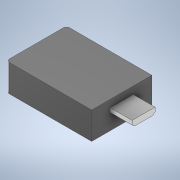
# Autodesk Inventor part: ND-105C
Saved by Autodesk Inventor 2020.2 (Build 242310000, 310)
## iProperties
Created: 2020-04-10
Part Number: ND-105C
Material: PC/ABS Plastic
Document SubType Name: Modeling
Designer: agmlego
Mass: 1.34202 g
Surface Area: 17.1017 cm^2
Volume: 3.75629 cm^3
Density: 0.357273 g/cm^3
Appearance: Smooth - Black
Author: agmlego
Autodesk Inventor part; units mm, degrees
ref_plane "YZ Plane" through (0, 0, 0) normal (1, 0, 0) x (0, 1, 0)
ref_plane "XZ Plane" through (0, 0, 0) normal (0, 1, 0) x (-1, 0, 0)
ref_plane "XY Plane" through (0, 0, 0) normal (0, 0, 1) x (1, 0, 0)
sketch "Sketch1" plane through (0, 0, 0) normal (0, 1, 0) x (-1, 0, 0)
  line L0 (0, 0) -> (25.4, 0)
  line L1 (25.4, 0) -> (25.4, -17.9)
  line L2 (25.4, -17.9) -> (0, -17.9)
  line L3 (0, -17.9) -> (0, 0)
  dimension "d0" = 25.4
  dimension "d1" = 17.9
  constraints: 8 end point, 2 parallel, 1 horizontal, 1 perpendicular
  measures "d0" distance of L0.start L0.end
  measures "d1" distance of L2.end L0.start
extrude "Extrusion1" add sketch "Sketch1" along normal blind 8.1
fillet "Fillet1" radius 1 2 edges at (-25.4, 4.05, 0) (-25.4, 4.05, -17.9)
sketch "Sketch2" plane through (0, 0, 0) normal (1, 0, 0) x (0, 0, -1)
  line L0 (5.53, 5.9) -> (12.37, 5.9)
  line L1 (12.37, 5.9) -> (12.37, 4.7)
  line L2 (12.37, 4.7) -> (11.6, 4.1)
  line L3 (11.6, 4.1) -> (6.3, 4.1)
  line L4 (6.3, 4.1) -> (5.53, 4.7)
  line L5 (5.53, 4.7) -> (5.53, 5.9)
  line L6 (8.95, 5.9) -> (8.95, 4.1) construction
  line L7 (0, 8.1) -> (17.9, 8.1) construction
  point P0 (0, 0)
  point P1 (8.95, 8.1)
  dimension "d5" = 2.2
  dimension "d6" = 6.84
  dimension "d7" = 1.8
  dimension "d8" = 1.2
  dimension "d9" = 5.3
  constraints: 14 end point, 3 midpoint, 2 equal length, 2 parallel, 1 horizontal, 1 perpendicular, 1 point on line
  measures "d5" distance between parallel lines of L7 L0
  measures "d6" distance between parallel lines of L1 L5
  measures "d7" distance of L6.start L6.end
  measures "d8" distance of L0.end L1.end
  measures "d9" distance of L2.end L3.end
extrude "Extrusion2" add sketch "Sketch2" along normal blind 6.5
body "Solid1"
